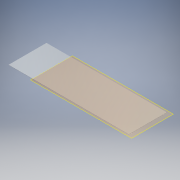
# Autodesk Inventor part: Part42
Saved by Autodesk Inventor 2016 (Build 200138000, 138)
## iProperties
Created: 2018-06-25
Part Number: Part42
Material: Glass
Document SubType Name: Modeling
Designer: damia
Density: 2.18 g/cm^3
Appearance: Clear
Mass: 5486.4 g
Surface Area: 12693.2 cm^2
Volume: 2516.7 cm^3
Author: damia
Autodesk Inventor part; units mm, degrees
ref_plane "YZ Plane" through (0, 0, 0) normal (1, 0, 0) x (0, 1, 0)
ref_plane "XZ Plane" through (0, 0, 0) normal (0, 1, 0) x (-1, 0, 0)
ref_plane "XY Plane" through (0, 0, 0) normal (0, 0, 1) x (1, 0, 0)
ref_plane "Work Plane1" through (318, -51, 0) normal (0, 0, 1) x (1, 0, 0)
sketch "Sketch1" plane through (318, -51, 0) normal (0, 0, 1) x (1, 0, 0)
  line L0 (407, 351) -> (-1175, 351) projected
  line L1 (-1175, 351) -> (-1175, -300) projected
  line L2 (-1175, -300) -> (407, -300) projected
  line L3 (407, -300) -> (407, 351) projected
  point P0 (-318, 51)
extrude "Extrusion1" add sketch "Sketch1" along normal blind 4
chamfer "Chamfer1" distance 1 angle 45 12 edges at (725, -25.5, 4) (-66, 300, 4) (725, 300, 2) (-66, 300, 0) (725, -25.5, 0) (725, -351, 2) (-66, -351, 4) (-66, -351, 0) (-857, -351, 2) (-857, -25.5, 0) (-857, -25.5, 4) (-857, 300, 2)
body "Solid1"
